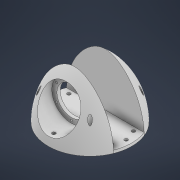
# Autodesk Inventor part: Bottom2
Saved by Autodesk Inventor 2021 (Build 250183000, 183)
## iProperties
Created: 2022-09-29
Part Number: Bottom2
Material: Ogólny
Document SubType Name: Modeling
Designer: MicnedSQ
Density: 1 g/cm^3
Appearance: Domyślna
Author: MicnedSQ
Autodesk Inventor part; units mm, degrees
sketch "Szkic1" plane through (0, 0, 0) normal (0, 1, 0) x (-1, 0, 0)
  circle A0 centre (0, 0) radius 75
  dimension "d0" = 150
  constraints: 1 centre point, 1 coincident
  measures "d0" diameter of A0
extrude "Wyciągnięcie proste1" add sketch "Szkic1" along normal blind 100
sketch "Szkic5" plane through (0, 0, 0) normal (1, 0, 0) x (0, 1, 0)
  line L0 (100, -75) -> (100, 75) projected
  line L1 (100, 27.5) -> (5, 27.5)
  line L2 (5, 27.5) -> (5, -27.5)
  line L3 (5, -27.5) -> (100, -27.5)
  line L4 (100, -27.5) -> (100, 27.5)
  point P0 (0, 0)
  point P1 (5, 0)
  dimension "d7" = 95
  dimension "d8" = 55
  constraints: 8 end point, 2 parallel, 1 horizontal, 1 horizontal alignment, 1 midpoint, 1 perpendicular, 1 point on line
  measures "d7" distance of L3.end L2.end
  measures "d8" distance of L2.end L1.end
extrude "Wyciągnięcie proste3" cut sketch "Szkic5" along normal mid plane 150
sketch "Szkic6" plane through (0, 0, 0) normal (1, 0, 0) x (0, 1, 0)
  line L0 (0, -75) -> (0, 75) projected
  arc A0 (100, 27.5) -> (0, 75) centre (0.0012, -54.0107) ccw
  line L1 (0, 75) -> (100, 75)
  line L2 (100, 75) -> (100, 27.5)
  line L3 (-21.0708, 0) -> (126.4249, 0) projected
  point P0 (0, 0)
  constraints: 4 end point, 2 point on circle, 1 centre point, 1 horizontal
revolve "Obrót1" cut sketch "Szkic6" angle 360 about axis through (0, -10, 0) along (0, 1, 0)
sketch "Szkic7" plane through (-69.3591, 5, 27.5) normal (0, 1, 0) x (1, 0, 0)
  line L0 (-0.3132, 0) -> (139.0313, 0) projected
  line L1 (139.0313, 55) -> (-0.3132, 55) projected
  point P0 (69.3591, 27.5)
  point P1 (0, 0)
  point P2 (138.7181, 0)
  point P3 (138.7181, 55)
  point P4 (0, 55)
  point P5 (11.3438, 7.5)
  point P6 (-8.406, 0)
  point P7 (91.594, 0)
  point P8 (91.594, 55)
  point P9 (-0.4174, 0)
  point P10 (139.1355, 0)
  point P11 (139.1355, 55)
  point P12 (-0.4174, 55)
hole "Otwór1" at (-58.0152, 5, 20) direction (0, -1, 0) diameter 3.5 end through all
sketch "Szkic8" plane through (-69.3591, 5, 27.5) normal (0, 1, 0) x (1, 0, 0)
  circle A0 centre (11.3438, 7.5) radius 1.75 projected
  circle A1 centre (11.3438, 7.5) radius 3
  point P0 (69.3591, 27.5)
  dimension "d20" = 6
  constraints: 1 centre point, 1 coincident
  measures "d20" diameter of A1
extrude "Wyciągnięcie proste4" cut sketch "Szkic8" against normal blind 4
mirror "Odbij1" about plane through (0, 0, 0) normal (0, 0, 1) of "Wyciągnięcie proste4", "Otwór1"
mirror "Odbij2" about plane through (0, 0, 0) normal (1, 0, 0) of "Wyciągnięcie proste4", "Otwór1", "Odbij1"
ref_plane "Płaszczyzna konstrukcyjna2" through (0, 0, 75) normal (0, 0, 1) x (1, 0, 0)
sketch "Szkic12" plane through (0, 0, 75) normal (0, 0, 1) x (1, 0, 0)
  circle A0 centre (0, 50) radius 35
  line L0 (75, 0) -> (-75, 0) projected
  point P0 (0, 0)
  dimension "d30" = 70
  dimension "d31" = 50
  constraints: 1 centre point
  measures "d30" diameter of A0
  measures "d31" distance from line of L0 A0.centre
extrude "Wyciągnięcie proste6" cut sketch "Szkic12" against normal blind 41.5
sketch "Szkic14" plane through (0, 50, 33.5) normal (0, 0, 1) x (1, 0, 0)
  circle A0 centre (0, 0) radius 26
  point P0 (0, -50)
  dimension "d34" = 52
  constraints: 1 centre point
  measures "d34" diameter of A0
extrude "Wyciągnięcie proste7" cut sketch "Szkic14" against normal up to surface (6 mm away)
sketch "Szkic17" plane through (0, 50, 33.5) normal (0, 0, 1) x (1, 0, 0)
  circle A0 centre (0, 30.5) radius 1.9
  circle A1 centre (0, 0) radius 26 projected
  point P0 (0, -50)
  dimension "d47" = 3.8
  dimension "d48" = 30.5
  constraints: 1 centre point
  measures "d47" diameter of A0
  measures "d48" distance of A1.centre A0.centre
extrude "Wyciągnięcie proste10" cut sketch "Szkic17" against normal blind 5 contours A0
pattern_circular "Szyk kołowy2" count 6 over 360 about axis through (0, 50, 33.5) along (0, 0, -1) of "Wyciągnięcie proste10"
sketch "Szkic18" plane through (0, 0, 0) normal (0, -1, 0) x (1, 0, 0)
  point P0 (0, 0)
ref_plane "Płaszczyzna konstrukcyjna3" through (0, 100, 0) normal (0, 1, 0) x (-1, 0, 0)
sketch "Szkic19" plane through (0, 100, 0) normal (0, 1, 0) x (-1, 0, 0)
  circle A0 centre (65, 0) radius 3
  point P0 (0, 0)
  dimension "d55" = 6
  dimension "d65" = 65
  constraints: 1 centre point
  measures "d55" diameter of A0
  measures "d65" distance of point (0, 0) A0.centre
extrude "Wyciągnięcie proste11" cut sketch "Szkic19" against normal blind 98
sketch "Szkic20" plane through (-65, 2, 0) normal (0, 1, 0) x (1, 0, 0)
  circle A0 centre (0, 0) radius 3 projected
  circle A1 centre (0, 0) radius 1.75
  point P0 (65, 0)
  dimension "d58" = 3.5
  constraints: 1 centre point, 1 coincident
  measures "d58" diameter of A1
extrude "Wyciągnięcie proste12" cut sketch "Szkic20" against normal up to surface (2 mm away) contours A1
pattern_circular "Szyk kołowy3" count 8 over 360 about axis through (0, 0.0012, 0) along (0, -1, 0) of "Wyciągnięcie proste11", "Wyciągnięcie proste12"
ref_plane "Płaszczyzna konstrukcyjna4" through (75, 0, 0) normal (1, 0, 0) x (0, 1, 0)
sketch "Szkic21" plane through (75, 0, 0) normal (1, 0, 0) x (0, 1, 0)
  line L0 (5, 27.5) -> (0, 27.5)
  point P0 (0, 0)
  constraints: 2 end point, 1 horizontal
split body "Podział1" sketch "Szkic21" result two bodies curves L0 first body at (15.5265, 23.343, -70.6771)
sketch "Szkic22" plane through (75, 0, 0) normal (1, 0, 0) x (0, 1, 0)
  line L0 (5, -27.5) -> (0, -27.5)
  point P0 (0, 0)
  constraints: 2 end point, 1 horizontal
split body "Podział2" sketch "Szkic22" result two bodies bodies 2 curves L0 first body at (-23.0158, 23.343, -68.6046)
